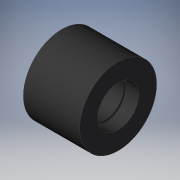
# Autodesk Inventor part: C-AFBD11-15_bw
Saved by Autodesk Inventor 2019 (Build 230136000, 136)
## iProperties
Created: 2023-11-09
Part Number: C-AFBD11-15_bw
Material: Generic
Catalog Web Link: www.cadenas.de
Description: C-AFBD-W, C-AFDF-W_bw-Economy Idlers Backside Tension Type
Vendor: MISUMI
Document SubType Name: Modeling
Designer: psAdmin
Manufacturer: MISUMI
Mass: 1.46163 g
Surface Area: 10.5243 cm^2
Volume: 1.46163 cm^3
Density: 1 g/cm^3
Appearance: PSOLRGB-175-175-175
Category: PARTsolutions
Company: MISUMI
Title: C-AFBD11-15
Author: Cadenas PARTsolutions
Comments: Economy Idlers Backside Tension Type
PSOL_IDENT_0: {$CADENAS_DATA/23d-libs/misumi/metric/51_timing_pulleys/c_afbd/c_afbd_w_body.prj},182 {VTYP=3D},{NB=
PSOL_IDENT_1: C-AFBD11-15_bw},{LINA=C-AFBD11-15},{NN=C-AFBD-W, C-AFDF-W_bw},{DATE=13.09.2022 06:55:24},{GEOMDATE=1
PSOL_IDENT_2: 8.05.2021 06:11:19},{VERSION=},{LINEID=30},{WBVAR=TS},{WBNUMERIC=}  {NB=C-AFBD11-15_bw},{LINA=C-AFBD
PSOL_IDENT_3: 11-15},{KT=DUMMY},{PN=C-AFBD11-15},{TYPE=C-AFBD},{TS=C-AFBD},{TSALG= 'C-AFBD','No Flange','C-AFDF','
PSOL_IDENT_4: Flanged' },{W=11},{NOM=15},{NOMALG= '15' },{D=15},{F=18},{A=7},{ABI=-},{ABM=60},{NO=675ZZ×2},{BN=675
PSOL_IDENT_5: },{DD=5},{B=2.5},{E=11.000},{BD=8.000},{DH=7.000},{PTT=1.000},{CIF=1.000}
NB: C-AFBD11-15_bw
NN: C-AFBD-W, C-AFDF-W_bw
NT: Economy Idlers Backside Tension Type
NBSYN: $PN._bw
LINA: C-AFBD11-15
CATALOG: Misumi
PN: C-AFBD11-15
TYPE: C-AFBD
TS: No Flange
W: 11
NOM: 15
D: 15
F: 18
A: 7
ABI: -
ABM: 60
NO: 675ZZ×2
BN: 675
DD: 5
B: 2.5
SUPPLIER: MISUMI
ARTICLENO: C-AFBD11-15_bw
BOMINFO: C-AFBD11-15
CREATOR: CADENAS GmbH
Autodesk Inventor part; units mm, degrees
sketch "_____1" plane through (0, 0, 0) normal (0, 0, 1) x (1, 0, 0)
  line L0 (5.5, 0) -> (-5.5, 0)
  line L1 (-5.5, 0) -> (-5.5, 7.5)
  line L2 (-5.5, 7.5) -> (5.5, 7.5)
  line L3 (5.5, 7.5) -> (5.5, 0)
  line L4 (5.5, 0) -> (-5.5, 0)
  constraints: 10 end point
revolve "Revolution1" add sketch "_____1" angle 360 about axis through (5.5, 0, 0) along (1, 0, 0)
sketch "_____3" plane through (0, 0, 0) normal (0, 0, 1) x (1, 0, 0)
  line L0 (5.5, 0) -> (-5.5, 0)
  line L1 (-5.5, 0) -> (-5.5, 4)
  line L2 (-5.5, 4) -> (-3, 4)
  line L3 (-3, 4) -> (-3, 3.5)
  line L4 (-3, 3.5) -> (3, 3.5)
  line L5 (3, 3.5) -> (3, 4)
  line L6 (3, 4) -> (5.5, 4)
  line L7 (5.5, 4) -> (5.5, 0)
  line L8 (5.5, 0) -> (-5.5, 0)
  constraints: 18 end point
revolve "Revolution2" cut sketch "_____3" angle 360 about axis through (5.5, 0, 0) along (1, 0, 0)
ref_plane "b600_1_XY" through (4.25, 0, 0) normal (1, 0, 0) x (0, 0, -1)
ref_plane "b600_1_YZ" through (4.25, 0, 0) normal (0, 0, -1) x (0, 1, 0)
ref_plane "b600_1_ZX" through (4.25, 0, 0) normal (0, 1, 0) x (1, 0, 0)
ref_plane "b600_2_XY" through (-4.25, 0, 0) normal (1, 0, 0) x (0, 0, -1)
ref_plane "b600_2_YZ" through (-4.25, 0, 0) normal (0, 0, -1) x (0, 1, 0)
ref_plane "b600_2_ZX" through (-4.25, 0, 0) normal (0, 1, 0) x (1, 0, 0)
ref_plane "to_dummy_XY" through (0, 0, 0) normal (1, 0, 0) x (0, 0, -1)
ref_plane "to_dummy_YZ" through (0, 0, 0) normal (0, 0, -1) x (0, 1, 0)
ref_plane "to_dummy_ZX" through (0, 0, 0) normal (0, 1, 0) x (1, 0, 0)
body "Solid1"
